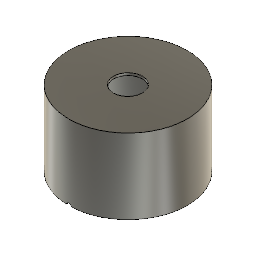
button (Autodesk Fusion 360 design; units mm, degrees)
part number: 2025-07-12-09-12-08-550
part number: 2025-07-12-12-01-52-056
part number: 2025-07-13-14-02-41-755
Autodesk Fusion 360 part; units mm, degrees
note: some values were not read from the file. Set by a fixed rule: which sketch regions a step uses.
sketch "Sketch2" plane through (0, 0, 0) normal (1, 0, 0) x (0, 1, 0) in component "tlacitko"
  line L0 (0, 0) -> (0, 84)
  line L1 (0, 0) -> (12, 0)
  line L2 (12, 0) -> (12, 37)
  line L3 (12, 37) -> (49, 37)
  line L4 (49, 37) -> (49, 54.5)
  spline S0 degree 5 poles (49, 54.5) (49.0182, 54.7054) (49.0464, 55.1092) (49.0636, 55.6937) (49.0363, 56.4305) (48.916, 57.2788) (48.706, 58.0532) (48.4023, 58.7534) (48.0013, 59.3822) (47.501, 59.9458) (46.9002, 60.4524) (46.1985, 60.911) (45.397, 61.3298) (44.4988, 61.7156) (43.5081, 62.0733) (42.4291, 62.4063) (41.4984, 62.6545) (40.7635, 62.831) (40.2572, 62.9444) (40, 63) knots 0 0 0 0 0 0 0.066667 0.133333 0.2 0.266667 0.333333 0.4 0.466667 0.533333 0.6 0.666667 0.733333 0.8 0.866667 0.933333 1 1 1 1 1 1
  spline S1 degree 5 poles (40, 63) (39.8948, 63.2852) (39.6672, 63.8526) (39.2736, 64.6949) (38.6446, 65.8003) (37.6848, 67.1519) (36.5554, 68.4714) (35.2658, 69.7555) (33.835, 70.999) (32.2897, 72.1951) (30.6607, 73.3373) (28.9791, 74.421) (27.2732, 75.4443) (25.5645, 76.4107) (23.866, 77.3285) (22.1838, 78.2071) (20.5175, 79.0548) (18.8613, 79.8756) (17.2044, 80.6658) (15.5326, 81.4135) (13.8295, 82.1015) (12.0789, 82.711) (10.2661, 83.2237) (8.3803, 83.6263) (6.4152, 83.9109) (4.3674, 84.0737) (2.6623, 84.1055) (1.3457, 84.0742) (0.4514, 84.0288) (0, 84) knots 0 0 0 0 0 0 0.04 0.08 0.12 0.16 0.2 0.24 0.28 0.32 0.36 0.4 0.44 0.48 0.52 0.56 0.6 0.64 0.68 0.72 0.76 0.8 0.84 0.88 0.92 0.96 1 1 1 1 1 1
  point P0 (48.4487, 58.5968)
  point P1 (46, 61)
  point P2 (36, 69)
  point P3 (28, 75)
  point P4 (19.4151, 79.5971)
  point P5 (11, 83)
  dimension "d14" = 12
  dimension "d15" = 17.5
  dimension "d42" = 37
  constraint coincident L0.start L1.start
  constraint vertical L0
  constraint perpendicular L0 L1
  constraint perpendicular L1 L2
  constraint perpendicular L2 L3
  constraint perpendicular L3 L4
  measures "d14" distance of L0.start L1.end
  measures "d15" distance of L3.end L4.end
  measures "d42" distance of L2.end L3.end
revolve "Revolve1" add sketch "Sketch2" angle 360 about axis through (0, 0, 0) along (0, 0, 1) makes body 1 in component "tlacitko"
sketch "Sketch2 (2)" plane through (0, 0, 0) normal (1, 0, 0) x (0, 1, 0) in component "zakladna"
  line L0 (-49, 37) -> (-12, 37)
  line L1 (-12, 37) -> (-12, 35)
  line L2 (-12, 35) -> (-49, 35)
  line L3 (-49, 35) -> (-49, 37)
  line L4 (-49, 35) -> (-47, 35)
  line L5 (-47, 35) -> (-47, -25)
  line L6 (-49, -25) -> (-49, 35)
  line L7 (-47, -25) -> (-49, -25)
  line L8 (-47, -25) -> (-42, -25)
  line L9 (-42, -25) -> (-42, -23)
  line L10 (-47, -23) -> (-47, -25)
  line L11 (-47, -18) -> (-47, -23)
  line L12 (-42, -23) -> (-47, -18)
  dimension "d20" = 37
  dimension "d21" = 2
  dimension "d22" = 2
  dimension "d23" = 60
  dimension "d40" = 49
  dimension "d41" = 25
  dimension "d43" = 2
  dimension "d44" = 5
  dimension "d45" = 5
  constraint horizontal L0
  constraint vertical L1
  constraint horizontal L2
  constraint vertical L3
  constraint horizontal L4
  constraint vertical L5
  constraint vertical L6
  constraint perpendicular L6 L7
  constraint horizontal L8
  constraint vertical L9
  constraint vertical L10
  constraint vertical L11
  measures "d20" distance of L0.start L0.end
  measures "d21" distance of L0.start L2.end
  measures "d22" distance of L2.end L4.end
  measures "d23" distance of L2.end L6.start
  measures "d40" distance of origin L6
  measures "d41" vertical distance of origin L6.start
  measures "d43" distance of L8.end L9.end
  measures "d44" distance of L5.end L8.end
  measures "d45" vertical distance of L9.end L11.start
revolve "Revolve2" add sketch "Sketch2 (2)" angle 360 about axis through (0, 0, 0) along (0, 0, 1) separate body makes body 2 in component "zakladna"
hole "Hole2" at (0, -49, -24.9998) direction (0, 1, 0) diameter 4 depth 10 tip angle 118 bodies 2 in component "zakladna"
component "tlacitko" placed x (1, 0, 0) y (0, 1, 0) z (0, 0, 1) at (0, 0, 0)
component "zakladna" placed x (1, 0, 0) y (0, 1, 0) z (0, 0, 1) at (0, 0, 0)
